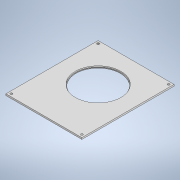
# Autodesk Inventor part: back
Saved by Autodesk Inventor 2021 (Build 250183000, 183)
## iProperties
Created: 2021-04-02
Part Number: back
Material: Generic
Document SubType Name: Modeling
Designer: awitc
Density: 1 g/cm^3
Appearance: Default
Author: awitc
Autodesk Inventor part; units mm, degrees
ref_plane "YZ Plane" through (0, 0, 0) normal (1, 0, 0) x (0, 1, 0)
ref_plane "XZ Plane" through (0, 0, 0) normal (0, 1, 0) x (-1, 0, 0)
ref_plane "XY Plane" through (0, 0, 0) normal (0, 0, 1) x (1, 0, 0)
sketch "Sketch1" plane through (0, 0, 0) normal (0, 1, 0) x (-1, 0, 0)
  line L0 (0, 0) -> (140, 0)
  line L1 (140, 0) -> (140, -170)
  line L2 (140, -170) -> (0, -170)
  line L3 (0, -170) -> (0, 0)
  line L4 (140, 0) -> (137.5, 0)
  line L5 (140, -2.5) -> (140, 0)
  line L6 (140, -170) -> (135, -170)
  line L7 (135, -170) -> (135, -165)
  line L8 (135, -165) -> (140, -165)
  line L9 (140, -165) -> (140, -170)
  circle A0 centre (135, -165) radius 2
  line L10 (0, 0) -> (5, 0)
  line L11 (5, 0) -> (5, -5)
  line L12 (5, -5) -> (0, -5)
  line L13 (0, -5) -> (0, 0)
  circle A1 centre (5, -5) radius 2
  circle A2 centre (5, -165) radius 2
  circle A3 centre (135, -5) radius 2
  dimension "d0" = 140
  dimension "d1" = 170
  dimension "d25" = 5
  dimension "d26" = 5
  dimension "d27" = 4
  dimension "d28" = 5
  dimension "d29" = 5
  dimension "d30" = 4
  dimension "d31" = 4
  dimension "d32" = 4
  constraints: 28 end point, 6 parallel, 4 centre point, 4 horizontal, 3 perpendicular, 2 coincident
  measures "d0" distance of L1.end L2.end
  measures "d1" distance of L0.end L1.end
  measures "d25" distance of L7.end L8.end
  measures "d26" distance of L6.end L7.end
  measures "d27" diameter of A0
  measures "d28" distance of L11.end L12.end
  measures "d29" distance of L10.end L11.end
  measures "d30" diameter of A1
  measures "d31" diameter of A2
  measures "d32" diameter of A3
extrude "Extrusion5" add sketch "Sketch1" along normal blind 3 contours L0 L11 A1 L12 L3 | L0 L1 L8 A0 L7 L2 L3 L12 A1 L11 | L7 A0 L8 L1 L2
sketch "Sketch5" plane through (0, 3, 0) normal (0, 1, 0) x (1, 0, 0)
  line L0 (0, 170) -> (-140, 170) projected
  circle A0 centre (-70, 100) radius 41
  point P0 (0, 0)
  dimension "d36" = 82
  constraints: 1 centre point
  measures "d36" diameter of A0
extrude "Extrusion6" cut sketch "Sketch5" against normal blind 10
sketch "Sketch6" plane through (0, 3, 0) normal (0, 1, 0) x (1, 0, 0)
  circle A0 centre (-70, 100) radius 41 projected
  circle A1 centre (-70, 100) radius 41
  circle A2 centre (-70, 100) radius 42
  point P0 (0, 0)
  dimension "d39" = 84
  constraints: 2 centre point, 2 coincident
  measures "d39" diameter of A2
extrude "Extrusion7" cut sketch "Sketch6" against normal blind 2
body "Solid1"
